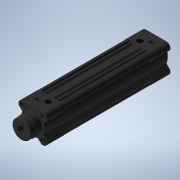
# Autodesk Inventor part: 1463250 DSBC-32-100-PPVA_(Z_0)
Saved by Autodesk Inventor 2021 (Build 250183000, 183)
## iProperties
Created: 2025-06-06
Part Number: 1463250 DSBC-32-100-PPVA_(Z_0)
Material: Generic
Catalog Web Link: www.cadenas.de
Description: DSBC_Z-Standard cylinder
Vendor: FESTO
Document SubType Name: Modeling
Designer: psAdmin
Manufacturer: FESTO
Mass: 206.246 g
Surface Area: 742.024 cm^2
Volume: 206.246 cm^3
Density: 1 g/cm^3
Appearance: PSOLRGB-175-175-175
Category: PARTsolutions
Company: FESTO
Title: 1463250 DSBC-100-PPVA_(Z_0)
Author: Cadenas PARTsolutions
Comments: Standard cylinder
PSOL_IDENT_0: {$CADENAS_DATA/23d-libs/festo/parts/d/dsbc/parts/dsbc_zyl.prj},244 {VTYP=3D},{NB=1463250 DSBC-32-100
PSOL_IDENT_1: -PPVA_(Z_0)},{LINA=1463250 DSBC-100-PPVA_(Z_0)},{NN=DSBC_Z},{DATE=30.04.2025 10:56:05},{GEOMDATE=16.
PSOL_IDENT_2: 09.2024 09:32:00},{VERSION=},{LINEID=10},{WBVAR=HUB,VER,END,DAE,DAEALG,KA,PRFA,TB,PAR},{WBNUMERIC=HU
PSOL_IDENT_3: B,DAEALG}  {NB=1463250 DSBC-32-100-PPVA_(Z_0)},{LINA=1463250 DSBC-100-PPVA_(Z_0)},{KT=DUMMY},{TNR=14
PSOL_IDENT_4: 63250},{TYP=DSBC},{KDM=32},{HUB=100},{HUBMAX=2800},{VER=-},{VER1='-','Q'},{VERT=},{END=-},{END1='-','
PSOL_IDENT_5: E1','E2','E3'},{ENDT=},{DAE=PPV},{DAE1='P','PPV','PPS'},{DAEALG=0},{KA=-},{KAT=},{PRFA=-},{PRFAT=},{
PSOL_IDENT_6: TB=-},{TBT=},{PAR=-},{PART=},{A1=35},{A2=500},{A=22},{AM=22},{AF=12},{B=30},{BA=30},{BG=16},{E=45},{
PSOL_IDENT_7: EE=G1/8},{EEK=9.728},{G=28.0},{J=28.0},{H1=5},{KF=M6},{KFK=6.000},{KK=M10x1.25},{KKDM=10.000},{KKP=1
PSOL_IDENT_8: .250},{L2=18.0},{L3=4.0},{L7=6.5},{L8N=94.000},{L8=194.000},{MM=12},{PL=19.5},{RT=M6},{RTK=6.000},{T
PSOL_IDENT_9: G=32.5},{U1=5.25},{U2=5.70},{VA=4},{VD=10.0},{W1=6.5},{W20=2.6},{WH=26.0},{WL=6.0},{ZJN=119.100},{ZJ=
PSOL_IDENT_10: 219.100},{ZMN=146.100},{ZM=346.100},{SW1=10},{SW2=16},{SW3=6},{D1=6.4},{D2=9.000},{D3=9.500},{T1=16.
PSOL_IDENT_11: 0},{T2=2.6},{R1=6.250},{R2=36.500},{B1=29.000},{L10=12.500},{L11=10.000},{L12=17.200},{L13=8.800},{L
PSOL_IDENT_12: 14=21.000},{L16=18.700},{L18=5.500},{SW6=6.000},{M1=6.000},{ANG=30.000},{D100=7.400},{L100=0.300},{B
PSOL_IDENT_13: E1=10.000},{E1=11.500},{HE=2.100},{HU=17.750},{LU=13.700},{RK=0.500},{RI=18.000},{R1I=6.000},{QH=10.
PSOL_IDENT_14: 000},{QR=1.000},{L101=0.000},{L102=0.000},{EB=46.500},{D3E=44.500},{RD3=45.000},{WD3=12.500},{D3HU1=
PSOL_IDENT_15: 17.750},{D3HU2=18.800},{D3X=41.500},{D3Y=31.000},{L4=14.000},{L5=14.000},{LD1=13.000},{LD2=3.000},{L
PSOL_IDENT_16: H1=57.500},{FDTB1DAMT=30},{L103=0.000},{HY1=0.000},{LX1=0.000},{LU2=13.700},{D3HU3=4.500},{LX2=0.000
PSOL_IDENT_17: },{HY2=0.000},{LX3=0.000},{RI2=18.000}
NB: 1463250 DSBC-32-100-PPVA_(Z_0)
NN: DSBC_Z
NT: Standard cylinder
NBSYN: $TNR. $TYP.-$KDM.$VERT.$ENDT.-$HUB.$KAT.$PRFAT.$TBT.$PART.-$DAE.A_(Z_$DAEALG.)
LINA: 1463250 DSBC-100-PPVA_(Z_0)
CATALOG: Festo
TNR: 1463250
TYP: DSBC
KDM: 32
HUB: 100
HUBMAX: 2800
VER: -
VER1: '-','Q'
END: -
DAE: PPV
DAE1: 'P','PPV','PPS'
DAEALG: 0
KA: -
PRFA: -
TB: -
PAR: -
A1: 35
A2: 500
A: 22
AM: 22
AF: 12
B: 30
BA: 30
BG: 16
E: 45
EE: G1/8
EEK: 9.728
G: 28
J: 28
H1: 5
KF: M6
KFK: 6
KK: M10x1.25
KKDM: 10
KKP: 1.25
L2: 18
L3: 4
L7: 6.5
L8N: 94
MM: 12
PL: 19.5
RT: M6
RTK: 6
TG: 32.5
U1: 5.25
U2: 5.7
VA: 4
VD: 10
W1: 6.5
W20: 2.6
WH: 26
WL: 6
ZJN: 119.1
ZMN: 146.1
SW1: 10
SW2: 16
SW3: 6
D1: 6.4
D2: 9
D3: 9.5
T1: 16
T2: 2.6
R1: 6.25
R2: 36.5
B1: 29
L10: 12.5
L11: 10
L12: 17.2
L13: 8.8
L14: 21
L16: 18.7
L18: 5.5
SW6: 6
M1: 6
ANG: 30
D100: 7.4
L100: 0.3
BE1: 10
E1: 11.5
HE: 2.1
HU: 17.75
LU: 13.7
RK: 0.5
RI: 18
R1I: 6
QH: 10
QR: 1
L101: 0
L102: 0
EB: 46.5
D3E: 44.5
RD3: 45
WD3: 12.5
D3HU1: 17.75
D3HU2: 18.8
D3X: 41.5
D3Y: 31
L4: 14
L5: 14
LD1: 13
LD2: 3
LH1: 57.5
FDTB1DAMT: 30
L103: 0
HY1: 0
LX1: 0
LU2: 13.7
D3HU3: 4.5
LX2: 0
HY2: 0
LX3: 0
RI2: 18
SUPPLIER: FESTO
ARTICLENO: 1463250 DSBC-32-100-PPVA_(Z_0)
BOMINFO: 1463250 DSBC-100-PPVA_(Z_0)
CREATOR: CADENAS GmbH
Autodesk Inventor part; units mm, degrees
ref_plane "YZ Plane" through (0, 0, 0) normal (1, 0, 0) x (0, 1, 0)
ref_plane "XZ Plane" through (0, 0, 0) normal (0, 1, 0) x (-1, 0, 0)
ref_plane "XY Plane" through (0, 0, 0) normal (0, 0, 1) x (1, 0, 0)
sketch "Sketch_1" plane through (0, 0, -28) normal (0, 0, 1) x (1, 0, 0)
  arc A0 (-22.5, 14.0754) -> (-22.2071, 13.3683) centre (-21.5, 14.0754) ccw
  line L0 (-22.2071, 13.3683) -> (-17.0289, 8.1901)
  arc A1 (-16.8147, 7.0943) -> (-17.0289, 8.1901) centre (-17.736, 7.483) ccw
  arc A2 (-16.8147, 7.0943) -> (-16.8147, -7.0943) centre (0, 0) ccw
  arc A3 (-17.0289, -8.1901) -> (-16.8147, -7.0943) centre (-17.736, -7.483) ccw
  line L1 (-17.0289, -8.1901) -> (-22.2071, -13.3683)
  arc A4 (-22.2071, -13.3683) -> (-22.5, -14.0754) centre (-21.5, -14.0754) ccw
  line L2 (-22.5, -14.0754) -> (-22.5, -16.25)
  arc A5 (-22.5, -16.25) -> (-16.25, -22.5) centre (-16.25, -16.25) ccw
  line L3 (-16.25, -22.5) -> (-14.0754, -22.5)
  arc A6 (-14.0754, -22.5) -> (-13.3683, -22.2071) centre (-14.0754, -21.5) ccw
  line L4 (-13.3683, -22.2071) -> (-8.1901, -17.0289)
  arc A7 (-7.0943, -16.8147) -> (-8.1901, -17.0289) centre (-7.483, -17.736) ccw
  arc A8 (-7.0943, -16.8147) -> (7.0943, -16.8147) centre (0, 0) ccw
  arc A9 (8.1901, -17.0289) -> (7.0943, -16.8147) centre (7.483, -17.736) ccw
  line L5 (8.1901, -17.0289) -> (13.3683, -22.2071)
  arc A10 (13.3683, -22.2071) -> (14.0754, -22.5) centre (14.0754, -21.5) ccw
  line L6 (14.0754, -22.5) -> (16.25, -22.5)
  arc A11 (16.25, -22.5) -> (22.5, -16.25) centre (16.25, -16.25) ccw
  line L7 (22.5, -16.25) -> (22.5, -14.0754)
  arc A12 (22.5, -14.0754) -> (22.2071, -13.3683) centre (21.5, -14.0754) ccw
  line L8 (22.2071, -13.3683) -> (17.0289, -8.1901)
  arc A13 (16.8147, -7.0943) -> (17.0289, -8.1901) centre (17.736, -7.483) ccw
  arc A14 (16.8147, -7.0943) -> (16.8147, 7.0943) centre (0, 0) ccw
  arc A15 (17.0289, 8.1901) -> (16.8147, 7.0943) centre (17.736, 7.483) ccw
  line L9 (17.0289, 8.1901) -> (22.2071, 13.3683)
  arc A16 (22.2071, 13.3683) -> (22.5, 14.0754) centre (21.5, 14.0754) ccw
  line L10 (22.5, 14.0754) -> (22.5, 16.25)
  arc A17 (22.5, 16.25) -> (16.25, 22.5) centre (16.25, 16.25) ccw
  line L11 (16.25, 22.5) -> (-16.25, 22.5)
  arc A18 (-16.25, 22.5) -> (-22.5, 16.25) centre (-16.25, 16.25) ccw
  line L12 (-22.5, 16.25) -> (-22.5, 14.0754)
  constraints: 38 point on circle, 26 end point, 19 centre point
extrude "Extrusion1" add sketch "Sketch_1" along normal blind 28
sketch "Sketch_8" plane through (0, 0, -28) normal (0, 0, 1) x (1, 0, 0)
  line L0 (-22.25, 13.7647) -> (-16.641, 8.1557)
  arc A0 (-16.5402, 7.5936) -> (-16.641, 8.1557) centre (-16.9946, 7.8022) ccw
  arc A1 (-16.5402, 7.5936) -> (-16.5402, -7.5936) centre (0, 0) ccw
  arc A2 (-16.641, -8.1557) -> (-16.5402, -7.5936) centre (-16.9946, -7.8022) ccw
  line L1 (-16.641, -8.1557) -> (-22.25, -13.7647)
  line L2 (-22.25, -13.7647) -> (-22.25, -16.25)
  arc A3 (-22.25, -16.25) -> (-16.25, -22.25) centre (-16.25, -16.25) ccw
  line L3 (-16.25, -22.25) -> (-13.7647, -22.25)
  line L4 (-13.7647, -22.25) -> (-8.1557, -16.641)
  arc A4 (-7.5936, -16.5402) -> (-8.1557, -16.641) centre (-7.8022, -16.9946) ccw
  arc A5 (-7.5936, -16.5402) -> (7.5936, -16.5402) centre (0, 0) ccw
  arc A6 (8.1557, -16.641) -> (7.5936, -16.5402) centre (7.8022, -16.9946) ccw
  line L5 (8.1557, -16.641) -> (13.7647, -22.25)
  line L6 (13.7647, -22.25) -> (16.25, -22.25)
  arc A7 (16.25, -22.25) -> (22.25, -16.25) centre (16.25, -16.25) ccw
  line L7 (22.25, -16.25) -> (22.25, -13.7647)
  line L8 (22.25, -13.7647) -> (16.641, -8.1557)
  arc A8 (16.5402, -7.5936) -> (16.641, -8.1557) centre (16.9946, -7.8022) ccw
  arc A9 (16.5402, -7.5936) -> (16.5402, 7.5936) centre (0, 0) ccw
  arc A10 (16.641, 8.1557) -> (16.5402, 7.5936) centre (16.9946, 7.8022) ccw
  line L9 (16.641, 8.1557) -> (22.25, 13.7647)
  line L10 (22.25, 13.7647) -> (22.25, 16.25)
  arc A11 (22.25, 16.25) -> (16.25, 22.25) centre (16.25, 16.25) ccw
  line L11 (16.25, 22.25) -> (-16.25, 22.25)
  arc A12 (-16.25, 22.25) -> (-22.25, 16.25) centre (-16.25, 16.25) ccw
  line L12 (-22.25, 16.25) -> (-22.25, 13.7647)
  constraints: 26 end point, 26 point on circle, 13 centre point
extrude "Extrusion2" add sketch "Sketch_8" against normal blind 138
sketch "Sketch_25" plane through (0, 0, -28) normal (0, 0, 1) x (1, 0, 0)
  line L0 (-27, -27) -> (27, -27)
  line L1 (27, -27) -> (27, 27)
  line L2 (27, 27) -> (-27, 27)
  line L3 (-27, 27) -> (-27, -27)
  arc A0 (-22.25, 15.4099) -> (-22.05, 15.0635) centre (-21.85, 15.4099) ccw
  line L4 (-22.05, 15.0635) -> (-20.288, 14.0462)
  arc A1 (-20.2051, 13.9826) -> (-20.288, 14.0462) centre (-20.488, 13.6997) ccw
  line L5 (-20.2051, 13.9826) -> (-15.7255, 9.503)
  arc A2 (-15.6445, 8.9022) -> (-15.7255, 9.503) centre (-16.0791, 9.1495) ccw
  arc A3 (-15.6445, 8.9022) -> (-15.6445, -8.9022) centre (0, 0) ccw
  arc A4 (-15.7255, -9.503) -> (-15.6445, -8.9022) centre (-16.0791, -9.1495) ccw
  line L6 (-15.7255, -9.503) -> (-20.2424, -14.0198)
  line L7 (-20.2424, -14.0198) -> (-22.05, -15.0635)
  arc A5 (-22.05, -15.0635) -> (-22.25, -15.4099) centre (-21.85, -15.4099) ccw
  line L8 (-22.25, -15.4099) -> (-22.25, -16.25)
  arc A6 (-22.25, -16.25) -> (-16.25, -22.25) centre (-16.25, -16.25) ccw
  line L9 (-16.25, -22.25) -> (-15.4099, -22.25)
  arc A7 (-15.4099, -22.25) -> (-15.0635, -22.05) centre (-15.4099, -21.85) ccw
  line L10 (-15.0635, -22.05) -> (-14.0462, -20.288)
  arc A8 (-13.9826, -20.2051) -> (-14.0462, -20.288) centre (-13.6997, -20.488) ccw
  line L11 (-13.9826, -20.2051) -> (-9.503, -15.7255)
  arc A9 (-8.9022, -15.6445) -> (-9.503, -15.7255) centre (-9.1495, -16.0791) ccw
  arc A10 (-8.9022, -15.6445) -> (8.9022, -15.6445) centre (0, 0) ccw
  arc A11 (9.503, -15.7255) -> (8.9022, -15.6445) centre (9.1495, -16.0791) ccw
  line L12 (9.503, -15.7255) -> (13.9826, -20.2051)
  arc A12 (14.0462, -20.288) -> (13.9826, -20.2051) centre (13.6997, -20.488) ccw
  line L13 (14.0462, -20.288) -> (15.0635, -22.05)
  arc A13 (15.0635, -22.05) -> (15.4099, -22.25) centre (15.4099, -21.85) ccw
  line L14 (15.4099, -22.25) -> (16.25, -22.25)
  arc A14 (16.25, -22.25) -> (22.25, -16.25) centre (16.25, -16.25) ccw
  line L15 (22.25, -16.25) -> (22.25, -15.4099)
  arc A15 (22.25, -15.4099) -> (22.05, -15.0635) centre (21.85, -15.4099) ccw
  line L16 (22.05, -15.0635) -> (20.2424, -14.0198)
  line L17 (20.2424, -14.0198) -> (15.7255, -9.503)
  arc A16 (15.6445, -8.9022) -> (15.7255, -9.503) centre (16.0791, -9.1495) ccw
  arc A17 (15.6445, -8.9022) -> (15.6445, 8.9022) centre (0, 0) ccw
  arc A18 (15.7255, 9.503) -> (15.6445, 8.9022) centre (16.0791, 9.1495) ccw
  line L18 (15.7255, 9.503) -> (20.2051, 13.9826)
  arc A19 (20.288, 14.0462) -> (20.2051, 13.9826) centre (20.488, 13.6997) ccw
  line L19 (20.288, 14.0462) -> (22.05, 15.0635)
  arc A20 (22.05, 15.0635) -> (22.25, 15.4099) centre (21.85, 15.4099) ccw
  line L20 (22.25, 15.4099) -> (22.25, 16.25)
  arc A21 (22.25, 16.25) -> (16.25, 22.25) centre (16.25, 16.25) ccw
  line L21 (16.25, 22.25) -> (15.4099, 22.25)
  arc A22 (15.4099, 22.25) -> (15.0635, 22.05) centre (15.4099, 21.85) ccw
  line L22 (15.0635, 22.05) -> (14.082, 20.35)
  arc A23 (13.7356, 20.15) -> (14.082, 20.35) centre (13.7356, 20.55) ccw
  line L23 (13.7356, 20.15) -> (13.4713, 20.15)
  arc A24 (12.4107, 20.5893) -> (13.4713, 20.15) centre (13.4713, 21.65) ccw
  line L24 (12.4107, 20.5893) -> (10.8672, 22.1328)
  arc A25 (10.8672, 22.1328) -> (10.5843, 22.25) centre (10.5843, 21.85) ccw
  line L25 (10.5843, 22.25) -> (9.85, 22.25)
  arc A26 (9.85, 22.25) -> (9.45, 21.85) centre (9.85, 21.85) ccw
  line L26 (9.45, 21.85) -> (9.45, 21.15)
  arc A27 (9.45, 21.15) -> (9.65, 20.95) centre (9.65, 21.15) ccw
  line L27 (9.65, 20.95) -> (9.9, 20.95)
  arc A28 (10.1, 20.75) -> (9.9, 20.95) centre (9.9, 20.75) ccw
  line L28 (10.1, 20.75) -> (10.1, 18.15)
  arc A29 (9.7, 17.75) -> (10.1, 18.15) centre (9.7, 18.15) ccw
  line L29 (9.7, 17.75) -> (4, 17.75)
  arc A30 (3.6, 18.15) -> (4, 17.75) centre (4, 18.15) ccw
  line L30 (3.6, 18.15) -> (3.6, 20.75)
  arc A31 (3.8, 20.95) -> (3.6, 20.75) centre (3.8, 20.75) ccw
  line L31 (3.8, 20.95) -> (4.05, 20.95)
  arc A32 (4.05, 20.95) -> (4.25, 21.15) centre (4.05, 21.15) ccw
  line L32 (4.25, 21.15) -> (4.25, 21.85)
  arc A33 (4.25, 21.85) -> (3.85, 22.25) centre (3.85, 21.85) ccw
  line L33 (3.85, 22.25) -> (-3.85, 22.25)
  arc A34 (-3.85, 22.25) -> (-4.25, 21.85) centre (-3.85, 21.85) ccw
  line L34 (-4.25, 21.85) -> (-4.25, 21.15)
  arc A35 (-4.25, 21.15) -> (-4.05, 20.95) centre (-4.05, 21.15) ccw
  line L35 (-4.05, 20.95) -> (-3.8, 20.95)
  arc A36 (-3.6, 20.75) -> (-3.8, 20.95) centre (-3.8, 20.75) ccw
  line L36 (-3.6, 20.75) -> (-3.6, 18.15)
  arc A37 (-4, 17.75) -> (-3.6, 18.15) centre (-4, 18.15) ccw
  line L37 (-4, 17.75) -> (-9.7, 17.75)
  arc A38 (-10.1, 18.15) -> (-9.7, 17.75) centre (-9.7, 18.15) ccw
  line L38 (-10.1, 18.15) -> (-10.1, 20.75)
  arc A39 (-9.9, 20.95) -> (-10.1, 20.75) centre (-9.9, 20.75) ccw
  line L39 (-9.9, 20.95) -> (-9.65, 20.95)
  arc A40 (-9.65, 20.95) -> (-9.45, 21.15) centre (-9.65, 21.15) ccw
  line L40 (-9.45, 21.15) -> (-9.45, 21.85)
  arc A41 (-9.45, 21.85) -> (-9.85, 22.25) centre (-9.85, 21.85) ccw
  line L41 (-9.85, 22.25) -> (-10.5843, 22.25)
  arc A42 (-10.5843, 22.25) -> (-10.8672, 22.1328) centre (-10.5843, 21.85) ccw
  line L42 (-10.8672, 22.1328) -> (-12.4107, 20.5893)
  arc A43 (-13.4713, 20.15) -> (-12.4107, 20.5893) centre (-13.4713, 21.65) ccw
  line L43 (-13.4713, 20.15) -> (-13.7356, 20.15)
  arc A44 (-14.082, 20.35) -> (-13.7356, 20.15) centre (-13.7356, 20.55) ccw
  line L44 (-14.082, 20.35) -> (-15.0635, 22.05)
  arc A45 (-15.0635, 22.05) -> (-15.4099, 22.25) centre (-15.4099, 21.85) ccw
  line L45 (-15.4099, 22.25) -> (-16.25, 22.25)
  arc A46 (-16.25, 22.25) -> (-22.25, 16.25) centre (-16.25, 16.25) ccw
  line L46 (-22.25, 16.25) -> (-22.25, 15.4099)
  constraints: 94 end point, 94 point on circle, 47 centre point
extrude "Extrusion3" cut sketch "Sketch_25" against normal blind 138
sketch "Sketch_51" plane through (0, 0, -194) normal (0, 0, 1) x (1, 0, 0)
  arc A0 (-22.5, 14.0754) -> (-22.2071, 13.3683) centre (-21.5, 14.0754) ccw
  line L0 (-22.2071, 13.3683) -> (-17.0289, 8.1901)
  arc A1 (-16.8147, 7.0943) -> (-17.0289, 8.1901) centre (-17.736, 7.483) ccw
  arc A2 (-16.8147, 7.0943) -> (-16.8147, -7.0943) centre (0, 0) ccw
  arc A3 (-17.0289, -8.1901) -> (-16.8147, -7.0943) centre (-17.736, -7.483) ccw
  line L1 (-17.0289, -8.1901) -> (-22.2071, -13.3683)
  arc A4 (-22.2071, -13.3683) -> (-22.5, -14.0754) centre (-21.5, -14.0754) ccw
  line L2 (-22.5, -14.0754) -> (-22.5, -16.25)
  arc A5 (-22.5, -16.25) -> (-16.25, -22.5) centre (-16.25, -16.25) ccw
  line L3 (-16.25, -22.5) -> (-14.0754, -22.5)
  arc A6 (-14.0754, -22.5) -> (-13.3683, -22.2071) centre (-14.0754, -21.5) ccw
  line L4 (-13.3683, -22.2071) -> (-8.1901, -17.0289)
  arc A7 (-7.0943, -16.8147) -> (-8.1901, -17.0289) centre (-7.483, -17.736) ccw
  arc A8 (-7.0943, -16.8147) -> (7.0943, -16.8147) centre (0, 0) ccw
  arc A9 (8.1901, -17.0289) -> (7.0943, -16.8147) centre (7.483, -17.736) ccw
  line L5 (8.1901, -17.0289) -> (13.3683, -22.2071)
  arc A10 (13.3683, -22.2071) -> (14.0754, -22.5) centre (14.0754, -21.5) ccw
  line L6 (14.0754, -22.5) -> (16.25, -22.5)
  arc A11 (16.25, -22.5) -> (22.5, -16.25) centre (16.25, -16.25) ccw
  line L7 (22.5, -16.25) -> (22.5, -14.0754)
  arc A12 (22.5, -14.0754) -> (22.2071, -13.3683) centre (21.5, -14.0754) ccw
  line L8 (22.2071, -13.3683) -> (17.0289, -8.1901)
  arc A13 (16.8147, -7.0943) -> (17.0289, -8.1901) centre (17.736, -7.483) ccw
  arc A14 (16.8147, -7.0943) -> (16.8147, 7.0943) centre (0, 0) ccw
  arc A15 (17.0289, 8.1901) -> (16.8147, 7.0943) centre (17.736, 7.483) ccw
  line L9 (17.0289, 8.1901) -> (22.2071, 13.3683)
  arc A16 (22.2071, 13.3683) -> (22.5, 14.0754) centre (21.5, 14.0754) ccw
  line L10 (22.5, 14.0754) -> (22.5, 16.25)
  arc A17 (22.5, 16.25) -> (16.25, 22.5) centre (16.25, 16.25) ccw
  line L11 (16.25, 22.5) -> (-16.25, 22.5)
  arc A18 (-16.25, 22.5) -> (-22.5, 16.25) centre (-16.25, 16.25) ccw
  line L12 (-22.5, 16.25) -> (-22.5, 14.0754)
  constraints: 38 point on circle, 26 end point, 19 centre point
extrude "Extrusion4" add sketch "Sketch_51" along normal blind 28
sketch "Sketch_3" plane through (0, 0, 0) normal (1, 0, 0) x (0, 1, 0)
  line L0 (0, 0) -> (0, 18)
  line L1 (0, 18) -> (13.8691, 18)
  line L2 (13.8691, 18) -> (14.3691, 17.5)
  line L3 (14.3691, 17.5) -> (14.4911, 10.5089)
  line L4 (14.4911, 10.5089) -> (15, 10)
  line L5 (15, 10) -> (15, 0)
  line L6 (15, 0) -> (0, 0)
  line L7 (0, 0) -> (0, 18)
  constraints: 16 end point
revolve "Revolution1" add sketch "Sketch_3" angle 360 about axis through (0, 0, 0) along (0, 0, -1)
sketch "Sketch6" plane through (-16.25, 22.5, -28) normal (0, 1, 0) x (1, 0, 0)
  point P0 (21.5, -8.5)
hole "Hole1" at (5.25, 22.5, -19.5) direction (0, -1, 0) diameter 8.566 depth 22.5 countersink diameter 9.728 countersink angle 90 thread size "G9.728x0.907" designation "G 1/8" standard "ISO Pipe Threads"
sketch "Sketch_4" plane through (-5.7, 0, 0) normal (1, 0, 0) x (0, 0, -1)
  line L0 (13, 18.5) -> (13, 22.5)
  line L1 (13, 22.5) -> (17.4, 22.5)
  line L2 (17.4, 22.5) -> (17.4, 22.2)
  line L3 (17.4, 22.2) -> (17.3015, 21.9295)
  arc A0 (17.3015, 21.9295) -> (17, 20.2194) centre (22, 20.2194) ccw
  line L4 (17, 20.2194) -> (17, 18.5)
  line L5 (17, 18.5) -> (13, 18.5)
  line L6 (13, 18.5) -> (13, 22.5)
  constraints: 14 end point, 2 point on circle, 1 centre point
revolve "Revolution2" cut sketch "Sketch_4" angle 360 about axis through (-5.7, 18.5, -13) along (0, -1, 0)
sketch "Sketch_45" plane through (-5.7, 0, 0) normal (1, 0, 0) x (0, 0, -1)
  line L0 (13, 17.5) -> (13, 20.7)
  line L1 (13, 20.7) -> (14.7295, 20.7)
  line L2 (14.7295, 20.7) -> (15.2295, 20.2)
  line L3 (15.2295, 20.2) -> (15.2295, 22.2295)
  line L4 (15.2295, 22.2295) -> (15.5, 22.5)
  line L5 (15.5, 22.5) -> (16.85, 22.5)
  line L6 (16.85, 22.5) -> (17, 22.2402)
  line L7 (17, 22.2402) -> (17, 17.5)
  line L8 (17, 17.5) -> (13, 17.5)
  line L9 (13, 17.5) -> (13, 20.7)
  constraints: 20 end point
revolve "Revolution3" add sketch "Sketch_45" angle 360 about axis through (-5.7, 17.5, -13) along (0, -1, 0)
thread "Thread1" size "M5x0.5" class "6H" standard "ISO Metric profile" full length
sketch "Sketch_48" plane through (-5.7, 20.7, -13) normal (0, 1, 0) x (0, 0, -1)
  line L0 (-0.4, -2) -> (0.4, -2)
  line L1 (0.4, -2) -> (0.4, 2)
  line L2 (0.4, 2) -> (-0.4, 2)
  line L3 (-0.4, 2) -> (-0.4, -2)
  constraints: 8 end point
extrude "Extrusion5" cut sketch "Sketch_48" against normal blind 1
sketch "Sketch_9" plane through (16.25, 0, 0) normal (1, 0, 0) x (0, 0, -1)
  line L0 (21, 16.25) -> (0, 16.25)
  line L1 (0, 16.25) -> (0, 21)
  line L2 (0, 21) -> (21, 21)
  line L3 (21, 21) -> (21, 16.25)
  line L4 (21, 16.25) -> (0, 16.25)
  constraints: 10 end point
revolve "Revolution4" cut sketch "Sketch_9" angle 360 about axis through (16.25, 16.25, -21) along (0, 0, -1)
pattern_linear "Rectangular Pattern1" count 2 spacing 32.5 along (-1, 0, 0) count 2 spacing 32.5 along (0, -1, 0) of "Revolution4"
sketch "Sketch_11" plane through (16.25, 0, 0) normal (1, 0, 0) x (0, 0, -1)
  line L0 (21, 16.25) -> (0, 16.25)
  line L1 (0, 16.25) -> (0, 20.1726)
  line L2 (0, 20.1726) -> (1, 20.75)
  line L3 (1, 20.75) -> (21, 20.75)
  line L4 (21, 20.75) -> (21, 16.25)
  line L5 (21, 16.25) -> (0, 16.25)
  constraints: 12 end point
revolve "Revolution5" add sketch "Sketch_11" angle 360 about axis through (16.25, 16.25, -21) along (0, 0, -1)
pattern_linear "Rectangular Pattern2" count 2 spacing 32.5 along (-1, 0, 0) count 2 spacing 32.5 along (0, -1, 0) of "Revolution5"
sketch "Sketch_13" plane through (16.25, 0, 0) normal (1, 0, 0) x (0, 0, -1)
  line L0 (20.1194, 16.25) -> (0, 16.25)
  line L1 (0, 16.25) -> (0, 19.95)
  line L2 (0, 19.95) -> (0.4041, 19.25)
  line L3 (0.4041, 19.25) -> (5.5, 19.25)
  line L4 (5.5, 19.25) -> (6.0415, 18.7085)
  line L5 (6.0415, 18.7085) -> (18.7, 18.7085)
  line L6 (18.7, 18.7085) -> (20.1194, 16.25)
  line L7 (20.1194, 16.25) -> (0, 16.25)
  constraints: 16 end point
revolve "Revolution6" cut sketch "Sketch_13" angle 360 about axis through (16.25, 16.25, -20.1194) along (0, 0, -1)
thread "Thread2" size "M6x1" class "6H" standard "ISO Metric profile" length 9.9585
sketch "Sketch_14" plane through (0, 0, 0) normal (0, 0, 1) x (1, 0, 0)
  line L0 (12.7859, 16.25) -> (13.25, 15.4462)
  line L1 (13.25, 15.4462) -> (13.25, 14.5179)
  line L2 (13.25, 14.5179) -> (14.0538, 14.0538)
  line L3 (14.0538, 14.0538) -> (14.5179, 13.25)
  line L4 (14.5179, 13.25) -> (15.4462, 13.25)
  line L5 (15.4462, 13.25) -> (16.25, 12.7859)
  line L6 (16.25, 12.7859) -> (17.0538, 13.25)
  line L7 (17.0538, 13.25) -> (17.9821, 13.25)
  line L8 (17.9821, 13.25) -> (18.4462, 14.0538)
  line L9 (18.4462, 14.0538) -> (19.25, 14.5179)
  line L10 (19.25, 14.5179) -> (19.25, 15.4462)
  line L11 (19.25, 15.4462) -> (19.7141, 16.25)
  line L12 (19.7141, 16.25) -> (19.25, 17.0538)
  line L13 (19.25, 17.0538) -> (19.25, 17.9821)
  line L14 (19.25, 17.9821) -> (18.4462, 18.4462)
  line L15 (18.4462, 18.4462) -> (17.9821, 19.25)
  line L16 (17.9821, 19.25) -> (17.0538, 19.25)
  line L17 (17.0538, 19.25) -> (16.25, 19.7141)
  line L18 (16.25, 19.7141) -> (15.4462, 19.25)
  line L19 (15.4462, 19.25) -> (14.5179, 19.25)
  line L20 (14.5179, 19.25) -> (14.0538, 18.4462)
  line L21 (14.0538, 18.4462) -> (13.25, 17.9821)
  line L22 (13.25, 17.9821) -> (13.25, 17.0538)
  line L23 (13.25, 17.0538) -> (12.7859, 16.25)
  constraints: 48 end point
extrude "Extrusion6" cut sketch "Sketch_14" along normal mid plane 8
pattern_linear "Rectangular Pattern3" count 2 spacing 32.5 along (-1, 0, 0) count 2 spacing 32.5 along (0, -1, 0) of "Revolution6"
pattern_linear "Rectangular Pattern4" count 2 spacing 32.5 along (-1, 0, 0) count 2 spacing 32.5 along (0, -1, 0) of "Extrusion6"
sketch "Sketch_22" plane through (0, 0, 0) normal (1, 0, 0) x (0, 1, 0)
  line L0 (0, -198) -> (0, -194)
  line L1 (0, -194) -> (15, -194)
  line L2 (15, -194) -> (15, -197.5)
  line L3 (15, -197.5) -> (14.5, -198)
  line L4 (14.5, -198) -> (0, -198)
  line L5 (0, -198) -> (0, -194)
  constraints: 12 end point
revolve "Revolution7" add sketch "Sketch_22" angle 360 about axis through (0, 0, -198) along (0, 0, -1)
sketch "Sketch15" plane through (-16.25, 22.5, -194) normal (0, 1, 0) x (1, 0, 0)
  point P0 (11, -19.5)
hole "Hole2" at (-5.25, 22.5, -174.5) direction (0, -1, 0) diameter 8.566 depth 22.5 countersink diameter 9.728 countersink angle 90 thread size "G9.728x0.907" designation "G 1/8" standard "ISO Pipe Threads"
sketch "Sketch_24" plane through (5.7, 0, 0) normal (1, 0, 0) x (0, 0, -1)
  line L0 (181, 18.5) -> (181, 22.5)
  line L1 (181, 22.5) -> (185.4, 22.5)
  line L2 (185.4, 22.5) -> (185.4, 22.2)
  line L3 (185.4, 22.2) -> (185.3015, 21.9295)
  arc A0 (185.3015, 21.9295) -> (185, 20.2194) centre (190, 20.2194) ccw
  line L4 (185, 20.2194) -> (185, 18.5)
  line L5 (185, 18.5) -> (181, 18.5)
  line L6 (181, 18.5) -> (181, 22.5)
  constraints: 14 end point, 2 point on circle, 1 centre point
revolve "Revolution8" cut sketch "Sketch_24" angle 360 about axis through (5.7, 18.5, -181) along (0, -1, 0)
sketch "Sketch_52" plane through (5.7, 0, 0) normal (1, 0, 0) x (0, 0, -1)
  line L0 (181, 17.5) -> (181, 20.7)
  line L1 (181, 20.7) -> (182.7295, 20.7)
  line L2 (182.7295, 20.7) -> (183.2295, 20.2)
  line L3 (183.2295, 20.2) -> (183.2295, 22.2295)
  line L4 (183.2295, 22.2295) -> (183.5, 22.5)
  line L5 (183.5, 22.5) -> (184.85, 22.5)
  line L6 (184.85, 22.5) -> (185, 22.2402)
  line L7 (185, 22.2402) -> (185, 17.5)
  line L8 (185, 17.5) -> (181, 17.5)
  line L9 (181, 17.5) -> (181, 20.7)
  constraints: 20 end point
revolve "Revolution9" add sketch "Sketch_52" angle 360 about axis through (5.7, 17.5, -181) along (0, -1, 0)
thread "Thread3" size "M5x0.5" class "6H" standard "ISO Metric profile" full length
sketch "Sketch_46" plane through (5.7, 20.7, -181) normal (0, 1, 0) x (0, 0, -1)
  line L0 (-0.4, -2) -> (0.4, -2)
  line L1 (0.4, -2) -> (0.4, 2)
  line L2 (0.4, 2) -> (-0.4, 2)
  line L3 (-0.4, 2) -> (-0.4, -2)
  constraints: 8 end point
extrude "Extrusion7" cut sketch "Sketch_46" against normal blind 1
sketch "Sketch19" plane through (0, 0, -194) normal (0, 0, -1) x (-1, 0, 0)
  point P0 (-16.25, 16.25)
hole "Hole3" at (16.25, 16.25, -194) direction (0, 0, 1) diameter 9.5 depth 21
pattern_linear "Rectangular Pattern5" count 2 spacing 32.5 along (-1, 0, 0) count 2 spacing 32.5 along (0, -1, 0) of "Hole3"
sketch "Sketch_30" plane through (16.25, 0, 0) normal (1, 0, 0) x (0, 0, -1)
  line L0 (194, 16.25) -> (173, 16.25)
  line L1 (173, 16.25) -> (173, 20.75)
  line L2 (173, 20.75) -> (193, 20.75)
  line L3 (193, 20.75) -> (194, 20.1726)
  line L4 (194, 20.1726) -> (194, 16.25)
  line L5 (194, 16.25) -> (173, 16.25)
  constraints: 12 end point
revolve "Revolution10" add sketch "Sketch_30" angle 360 about axis through (16.25, 16.25, -194) along (0, 0, -1)
pattern_linear "Rectangular Pattern6" count 2 spacing 32.5 along (-1, 0, 0) count 2 spacing 32.5 along (0, -1, 0) of "Revolution10"
sketch "Sketch_32" plane through (16.25, 0, 0) normal (1, 0, 0) x (0, 0, -1)
  line L0 (194, 16.25) -> (173.8806, 16.25)
  line L1 (173.8806, 16.25) -> (175.3, 18.7085)
  line L2 (175.3, 18.7085) -> (187.9585, 18.7085)
  line L3 (187.9585, 18.7085) -> (188.5, 19.25)
  line L4 (188.5, 19.25) -> (193.5959, 19.25)
  line L5 (193.5959, 19.25) -> (194, 19.95)
  line L6 (194, 19.95) -> (194, 16.25)
  line L7 (194, 16.25) -> (173.8806, 16.25)
  constraints: 16 end point
revolve "Revolution11" cut sketch "Sketch_32" angle 360 about axis through (16.25, 16.25, -194) along (0, 0, -1)
thread "Thread4" size "M6x1" class "6H" standard "ISO Metric profile" length 9.9585
pattern_linear "Rectangular Pattern7" count 2 spacing 32.5 along (-1, 0, 0) count 2 spacing 32.5 along (0, -1, 0) of "Revolution11"
sketch "Sketch_34" plane through (0, 0, -194) normal (0, 0, 1) x (1, 0, 0)
  line L0 (12.7859, 16.25) -> (13.25, 15.4462)
  line L1 (13.25, 15.4462) -> (13.25, 14.5179)
  line L2 (13.25, 14.5179) -> (14.0538, 14.0538)
  line L3 (14.0538, 14.0538) -> (14.5179, 13.25)
  line L4 (14.5179, 13.25) -> (15.4462, 13.25)
  line L5 (15.4462, 13.25) -> (16.25, 12.7859)
  line L6 (16.25, 12.7859) -> (17.0538, 13.25)
  line L7 (17.0538, 13.25) -> (17.9821, 13.25)
  line L8 (17.9821, 13.25) -> (18.4462, 14.0538)
  line L9 (18.4462, 14.0538) -> (19.25, 14.5179)
  line L10 (19.25, 14.5179) -> (19.25, 15.4462)
  line L11 (19.25, 15.4462) -> (19.7141, 16.25)
  line L12 (19.7141, 16.25) -> (19.25, 17.0538)
  line L13 (19.25, 17.0538) -> (19.25, 17.9821)
  line L14 (19.25, 17.9821) -> (18.4462, 18.4462)
  line L15 (18.4462, 18.4462) -> (17.9821, 19.25)
  line L16 (17.9821, 19.25) -> (17.0538, 19.25)
  line L17 (17.0538, 19.25) -> (16.25, 19.7141)
  line L18 (16.25, 19.7141) -> (15.4462, 19.25)
  line L19 (15.4462, 19.25) -> (14.5179, 19.25)
  line L20 (14.5179, 19.25) -> (14.0538, 18.4462)
  line L21 (14.0538, 18.4462) -> (13.25, 17.9821)
  line L22 (13.25, 17.9821) -> (13.25, 17.0538)
  line L23 (13.25, 17.0538) -> (12.7859, 16.25)
  constraints: 48 end point
extrude "Extrusion8" cut sketch "Sketch_34" along normal mid plane 8
pattern_linear "Rectangular Pattern8" count 2 spacing 32.5 along (-1, 0, 0) count 2 spacing 32.5 along (0, -1, 0) of "Extrusion8"
sketch "Sketch_42" plane through (0, 0, 0) normal (1, 0, 0) x (0, 1, 0)
  line L0 (0, -166) -> (0, 18)
  line L1 (0, 18) -> (6, 18)
  line L2 (6, 18) -> (6, -55.3333)
  line L3 (6, -55.3333) -> (16, -55.3333)
  line L4 (16, -55.3333) -> (16, -166)
  line L5 (16, -166) -> (0, -166)
  line L6 (0, -166) -> (0, 18)
  constraints: 14 end point
revolve "Revolution12" cut sketch "Sketch_42" angle 360 about axis through (0, 0, -166) along (0, 0, -1)
ref_plane "2DUMMY_XY" through (0, 0, 0) normal (0, 0, -1) x (1, 0, 0)
ref_plane "2DUMMY_YZ" through (0, 0, 0) normal (1, 0, 0) x (0, -1, 0)
ref_plane "2DUMMY_ZX" through (0, 0, 0) normal (0, -1, 0) x (0, 0, -1)
ref_plane "2P_XY" through (0, 0, -166) normal (0, 0, 1) x (1, 0, 0)
ref_plane "2P_YZ" through (0, 0, -166) normal (1, 0, 0) x (0, 1, 0)
ref_plane "2P_ZX" through (0, 0, -166) normal (0, 1, 0) x (0, 0, 1)
ref_plane "FDT_FRONT_XY" through (0, 0, 0) normal (0, 0, 1) x (1, 0, 0)
ref_plane "FDT_FRONT_YZ" through (0, 0, 0) normal (1, 0, 0) x (0, 1, 0)
ref_plane "FDT_FRONT_ZX" through (0, 0, 0) normal (0, 1, 0) x (0, 0, 1)
ref_plane "FDT_QSFRONT_XY" through (5.25, 22.5, -19.5) normal (0, 1, 0) x (1, 0, 0)
ref_plane "FDT_QSFRONT_YZ" through (5.25, 22.5, -19.5) normal (1, 0, 0) x (0, 0, -1)
ref_plane "FDT_QSFRONT_ZX" through (5.25, 22.5, -19.5) normal (0, 0, -1) x (0, 1, 0)
ref_plane "FDT_QSREAR_XY" through (-5.25, 22.5, -174.5) normal (0, 1, 0) x (1, 0, 0)
ref_plane "FDT_QSREAR_YZ" through (-5.25, 22.5, -174.5) normal (1, 0, 0) x (0, 0, -1)
ref_plane "FDT_QSREAR_ZX" through (-5.25, 22.5, -174.5) normal (0, 0, -1) x (0, 1, 0)
ref_plane "FDT_REAR_XY" through (0, 0, -194) normal (0, 0, 1) x (1, 0, 0)
ref_plane "FDT_REAR_YZ" through (0, 0, -194) normal (1, 0, 0) x (0, 1, 0)
ref_plane "FDT_REAR_ZX" through (0, 0, -194) normal (0, 1, 0) x (0, 0, 1)
ref_plane "FDT_SLOT1_XY" through (6.85, 17.75, -97) normal (0, 1, 0) x (1, 0, 0)
ref_plane "FDT_SLOT1_YZ" through (6.85, 17.75, -97) normal (1, 0, 0) x (0, 0, -1)
ref_plane "FDT_SLOT1_ZX" through (6.85, 17.75, -97) normal (0, 0, -1) x (0, 1, 0)
ref_plane "FDT_SLOT2_XY" through (-6.85, 17.75, -97) normal (0, 1, 0) x (1, 0, 0)
ref_plane "FDT_SLOT2_YZ" through (-6.85, 17.75, -97) normal (1, 0, 0) x (0, 0, -1)
ref_plane "FDT_SLOT2_ZX" through (-6.85, 17.75, -97) normal (0, 0, -1) x (0, 1, 0)
ref_plane "FDT_TRUNNMOUNT_XY" through (0, 0, -43) normal (0, 0, 1) x (1, 0, 0)
ref_plane "FDT_TRUNNMOUNT_YZ" through (0, 0, -43) normal (1, 0, 0) x (0, 1, 0)
ref_plane "FDT_TRUNNMOUNT_ZX" through (0, 0, -43) normal (0, 1, 0) x (0, 0, 1)
ref_plane "TO_C_XY" through (0, 0, -194) normal (0, 0, 1) x (1, 0, 0)
ref_plane "TO_C_YZ" through (0, 0, -194) normal (1, 0, 0) x (0, 1, 0)
ref_plane "TO_C_ZX" through (0, 0, -194) normal (0, 1, 0) x (0, 0, 1)
ref_plane "TO_P2_XY" through (0, 0, 18) normal (0, 0, 1) x (1, 0, 0)
ref_plane "TO_P2_YZ" through (0, 0, 18) normal (1, 0, 0) x (0, 1, 0)
ref_plane "TO_P2_ZX" through (0, 0, 18) normal (0, 1, 0) x (0, 0, 1)
body "Solid1"
